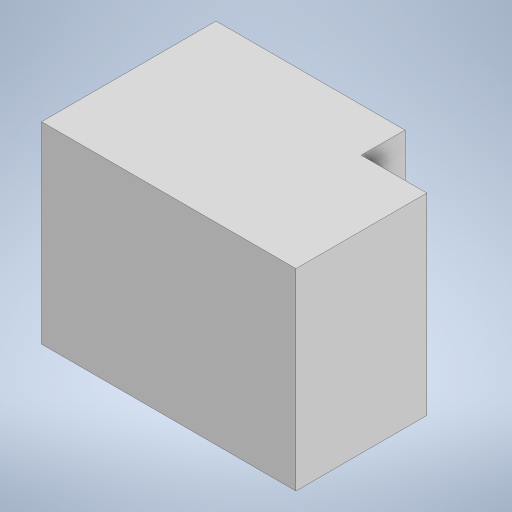
# Autodesk Inventor part: air
Saved by Autodesk Inventor 2023 (Build 270158000, 158)
## iProperties
Created: 2022-09-12
Part Number: air
Material: 常规
Document SubType Name: Modeling
Designer: byfbi
Density: 1 g/cm^3
Appearance: 默认
Author: byfbi
Autodesk Inventor part; units mm, degrees
ref_plane "YZ Plane" through (0, 0, 0) normal (1, 0, 0) x (0, 1, 0)
ref_plane "XZ Plane" through (0, 0, 0) normal (0, 1, 0) x (-1, 0, 0)
ref_plane "XY Plane" through (0, 0, 0) normal (0, 0, 1) x (1, 0, 0)
sketch "草图1" plane through (0, 0, 0) normal (0, 1, 0) x (-1, 0, 0)
  line L0 (0, 0) -> (0, 2400)
  line L1 (0, 2400) -> (-3500, 2400)
  line L2 (-3500, 2400) -> (-3500, 600)
  line L3 (-3500, 600) -> (-2600, 600)
  line L4 (-2600, 600) -> (-2600, 0)
  line L5 (-2600, 0) -> (0, 0)
  dimension "d0" = 2400
  dimension "d1" = 3500
  dimension "d2" = 1800
  dimension "d3" = 900
  constraints: 12 end point, 4 perpendicular, 1 horizontal, 1 vertical
  measures "d0" distance of L0.start L0.end
  measures "d1" distance of L0.end L1.end
  measures "d2" distance of L1.end L2.end
  measures "d3" distance of L2.end L3.end
extrude "拉伸1" add sketch "草图1" along normal blind 2650
